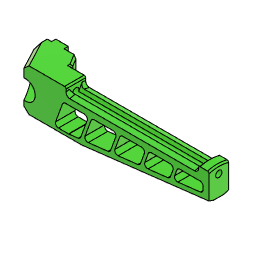
Single Piece Spool Holder v27 (Autodesk Fusion 360 design; units mm, degrees)
Autodesk Fusion 360 part; units mm, degrees
sketch "Sketch1" plane through (0, 0, 0) normal (0, 1, 0) x (1, 0, 0)
  line L0 (0, 0) -> (132, 0)
  line L1 (132, 0) -> (132, -30)
  line L2 (132, -30) -> (0, -30)
  line L3 (0, -30) -> (0, 0)
  line L4 (10, -30) -> (10, 0) construction
  line L5 (25, -30) -> (25, 0) construction
  dimension "d2" = 30
  dimension "d39" = 10
  dimension "d40" = 15
  dimension "d109" = 107
  constraint horizontal L0
  constraint vertical L1
  constraint horizontal L2
  constraint vertical L3
  constraint coincident L0.start L3.end
  constraint coincident L2 L4.start
  constraint coincident L0 L4.end
  constraint perpendicular L0 L4
  constraint coincident L2 L5.start
  constraint coincident L0 L5.end
  constraint perpendicular L0 L5
  measures "d2" distance of L0.start L2.end
  measures "d39" distance of L3 L4
  measures "d40" distance of L4 L5
  measures "d109" distance of L1 L5
extrude "Extrude1" add sketch "Sketch1" along normal mid plane 13 makes body 1
sketch "Sketch7" plane through (0, 6.5, 0) normal (0, 1, 0) x (-1, 0, 0)
  line L0 (0, 30) -> (-132, 30)
  line L1 (-132, 30) -> (-132, 0)
  line L2 (-132, 0) -> (0, 0)
  line L3 (0, 0) -> (0, 30)
  line L4 (0, 30) -> (-25, 30)
  line L5 (-25, 30) -> (-25, 0)
  line L6 (-25, 0) -> (0, 0)
  line L7 (0, 0) -> (0, 30)
  dimension "d75" = 25
  constraint horizontal L4
  constraint vertical L5
  constraint horizontal L6
  constraint vertical L7
  constraint coincident L2 L5.end
  constraint coincident L0.start L3.end
  measures "d75" distance of L0.start L4.end
extrude "Extrude9" add sketch "Sketch7" along normal blind 8.5 contours L0 L2 L3 L4 L5 L6 L7 bodies 1
sketch "Sketch2" plane through (0, 0, 0) normal (0, 0, 1) x (1, 0, 0)
  line L0 (0, -6.5) -> (0, 15)
  line L1 (25, 6.5) -> (132, 6.5)
  line L2 (132, 6.5) -> (132, -6.5)
  line L3 (132, -6.5) -> (0, -6.5)
  line L4 (5.825, 15) -> (14.175, 15)
  line L5 (14.175, 15) -> (14.175, 17.8)
  line L6 (14.175, 17.8) -> (5.825, 17.8)
  line L7 (5.825, 17.8) -> (5.825, 15)
  line L8 (10, 17.8) -> (10, 15) construction
  line L9 (0, 15) -> (25, 15)
  line L10 (25, 15) -> (25, 6.5)
  dimension "d20" = 10
  dimension "d21" = 2.8
  dimension "d22" = 8.35
  constraint horizontal L4
  constraint vertical L5
  constraint horizontal L6
  constraint vertical L7
  constraint midpoint L6 L8.start
  constraint midpoint L4 L8.end
  constraint coincident L9 L4.start
  constraint coincident L4.start L7.end
  measures "d20" distance of L0.end L8
  measures "d21" distance of L4.end L5.end
  measures "d22" distance of L5.end L6.end
extrude "Extrude2" add sketch "Sketch2" along normal blind 30 contours L4 L5 L6 L7 L9 bodies 1
sketch "Sketch3" plane through (0, -6.5, 0) normal (0, -1, 0) x (-1, 0, 0)
  line L0 (-10, -30) -> (-10, 0) construction
  circle A0 centre (-10, -15) radius 3.25
  line L1 (-132, -30) -> (0, -30)
  line L2 (0, -30) -> (0, 0)
  line L3 (0, 0) -> (-132, 0)
  line L4 (-132, 0) -> (-132, -30)
  line L5 (-14.175, 0) -> (-5.825, 0)
  line L6 (-5.825, 0) -> (-5.825, -30)
  line L7 (-5.825, -30) -> (-14.175, -30)
  line L8 (-14.175, -30) -> (-14.175, 0)
  dimension "d14" = 6.5
  constraint midpoint L0 A0.centre
  constraint midpoint L0.start L7
  constraint midpoint L0.end L5
  measures "d14" diameter of A0
extrude "Extrude3" cut sketch "Sketch3" against normal through all contours A0 bodies 1
sketch "Sketch4" plane through (0, -6.5, 0) normal (0, -1, 0) x (-1, 0, 0)
  circle A0 centre (-10, -15) radius 6.5
  circle A1 centre (-10, -15) radius 3.25
  line L0 (-132, -30) -> (0, -30)
  line L1 (0, -30) -> (0, 0)
  line L2 (0, 0) -> (-132, 0)
  line L3 (-132, 0) -> (-132, -30)
  dimension "d16" = 13
  constraint coincident A0.centre A1.centre
  measures "d16" diameter of A0
extrude "Extrude4" cut sketch "Sketch4" against normal up to surface (16 mm away) contours A0 | A1 bodies 1
chamfer "Chamfer1" distance 3.25 angle 45 1 edges at (13.0301, 9.5, 16.1753) on bodies 1
ref_plane "WorkPlane1" through (66, 5.65, 15) normal (0, 0, 1) x (1, 0, 0)
sketch "Sketch5" plane through (132, 0, 0) normal (1, 0, 0) x (0, 1, 0)
  line L0 (-6.5, 0) -> (6.5, 0)
  line L1 (6.5, 0) -> (6.5, 30)
  line L2 (6.5, 30) -> (-6.5, 30)
  line L3 (-6.5, 30) -> (-6.5, 0)
  circle A0 centre (0, 5.7) radius 20
  circle A1 centre (0, 5.7) radius 24
  line L4 (0, 0) -> (0, 30) construction
  circle A2 centre (0, 24.4) radius 2.1
  line L5 (-6.5, 0) -> (6.5, 0)
  line L6 (6.5, 0) -> (6.5, 30)
  line L7 (6.5, 30) -> (-6.5, 30)
  line L8 (-6.5, 30) -> (-6.5, 0)
  point P0 (27.1204, 5.059)
  point P1 (24.0412, 4.3321)
  point P2 (14.8796, 5.059)
  point P3 (17.9588, 4.3321)
  dimension "d86" = 40
  dimension "d87" = 48
  dimension "d88" = 5.7
  dimension "d89" = 24.4
  dimension "d90" = 4.2
  constraint coincident L4.start origin
  constraint midpoint L2 L4.end
  constraint coincident A0.centre A1.centre
  constraint coincident A0.centre L4
  constraint coincident L4 A2.centre
  measures "d86" diameter of A0
  measures "d87" diameter of A1
  measures "d88" distance of L0 A0.centre
  measures "d89" distance of L4.start A2.centre
  measures "d90" diameter of A2
extrude "Extrude5" cut sketch "Sketch5" against normal up to surface (88 mm away) from surface at -7 contours L1 L3 A0 A1 A2 L6 L8 | L1 L2 L3 A1 L6 L7 L8 | A0 A2 picked at (-0.0509, 25.9594) bodies 1
extrude "Extrude6" cut sketch "Sketch5" against normal blind 7 contours L1 L2 L3 A1 L6 L7 L8 bodies 1
extrude "Extrude7" cut sketch "Sketch5" against normal up to surface (102 mm away) contours A0 A2 | A0 A2 bodies 1
chamfer "Chamfer2" distance 1.3 distance2 2.2 2 edges at (81, -1.7041, 25.6273) (81, 1.7041, 25.6273) measured on face at (66.3333, -5.4581, 24.9408) measured on face at (66.3333, 2.2474, 25.5733) on bodies 1
fillet "Fillet1" radius 1 3 edges at (132, 0, 29.7) (125, 0, 29.7) (37, 0, 30) on bodies 1
chamfer "Chamfer3" distance 3 distance2 6 2 edges at (0, 4.25, 30) (0, 4.25, 0) measured on face at (20.3333, -2.1667, 30) measured on face at (52.3333, -2.1667, 0) on bodies 1
chamfer "Chamfer4" distance 11 distance2 93 1 edges at (132, 0, 0) measured on face at (132, 0.0523, 7.4353) on bodies 1
sketch "Sketch6" plane through (0, -6.5, 0) normal (0, -1, 0) x (1, 0, 0)
  line L0 (37, 24.6143) -> (37, 29)
  line L1 (36, 30) -> (3, 30)
  line L2 (3, 30) -> (0, 24)
  line L3 (0, 24) -> (0, 6)
  line L4 (0, 6) -> (3, 0)
  line L5 (3, 0) -> (39, 0)
  circle A0 centre (10, 15) radius 6.5
  line L6 (38.5445, 30) -> (27.6254, 0)
  line L7 (36.4161, 30) -> (25.497, 0)
  line L8 (0, 0) -> (128.5239, 0)
  line L9 (128.5239, 0) -> (128.5239, 30)
  line L10 (128.5239, 30) -> (0, 30)
  line L11 (0, 30) -> (0, 0)
  line L12 (55.4161, 30) -> (44.497, 0)
  line L13 (57.5445, 30) -> (46.6254, 0)
  line L14 (74.4161, 30) -> (63.497, 0)
  line L15 (76.5445, 30) -> (65.6254, 0)
  line L16 (93.4161, 30) -> (82.497, 0)
  line L17 (95.5445, 30) -> (84.6254, 0)
  line L18 (112.4161, 30) -> (101.497, 0)
  line L19 (114.5445, 30) -> (103.6254, 0)
  arc A1 (37, 29) -> (36, 30) centre (36, 29) ccw
  line L20 (39, 0) -> (132, 11)
  line L21 (132, 11) -> (132, 27.7624)
  spline S0 degree 3 poles (131, 28.803) (131.1219, 28.803) (131.2652, 28.7737) (131.4918, 28.6777) (131.6147, 28.5932) (131.7906, 28.4132) (131.8738, 28.285) (131.9704, 28.0461) (132, 27.8927) (132, 27.7624) knots 0.605058 0.605058 0.605058 0.605058 0.64162 0.64162 0.678904 0.678904 0.71712 0.71712 0.756197 0.756197 0.756197 0.756197
  line L22 (131, 28.803) -> (126, 28.803)
  spline S1 degree 3 poles (125, 27.7624) (125, 27.8927) (125.0296, 28.0461) (125.1262, 28.285) (125.2094, 28.4132) (125.3853, 28.5932) (125.5082, 28.6777) (125.7348, 28.7737) (125.8781, 28.803) (126, 28.803) knots 0.453919 0.453919 0.453919 0.453919 0.492996 0.492996 0.531212 0.531212 0.568496 0.568496 0.605058 0.605058 0.605058 0.605058
  line L23 (125, 27.7624) -> (125, 24.6143)
  line L24 (125, 24.6143) -> (37, 24.6143)
  line L25 (128, 14.5548) -> (128, 20.6143)
  line L26 (128, 20.6143) -> (33, 20.6143)
  line L27 (33, 20.6143) -> (33, 26)
  line L28 (33, 26) -> (5.4721, 26)
  line L29 (5.4721, 26) -> (4, 23.0557)
  line L30 (4, 23.0557) -> (4, 6.9443)
  line L31 (4, 6.9443) -> (5.4721, 4)
  line L32 (5.4721, 4) -> (38.7643, 4)
  line L33 (38.7643, 4) -> (128, 14.5548)
  line L34 (25, 30) -> (25, 0)
  line L35 (125, 22.6143) -> (35, 22.6143)
  line L36 (35, 22.6143) -> (35, 29)
  dimension "d51" = 2
  dimension "d55" = 76
  dimension "d56" = 0
  dimension "d59" = 30
  dimension "d61" = 70
  dimension "d101" = -4
  dimension "d108" = -2
  constraint parallel L6 L7
  constraint horizontal L8
  constraint vertical L9
  constraint horizontal L10
  constraint vertical L11
  constraint coincident L8.start L11.end
  constraint coincident L7.start L10
  constraint coincident L6.start L10
  constraint coincident L7.end L8
  constraint coincident L6.end L8
  constraint coincident L7 L26.end
  measures "d51" distance of L6 L7
  measures "d59" distance of L8 L10
  measures "d61" angle of L7 L10
extrude "Extrude8" cut sketch "Sketch6" against normal blind 47 contours L6 L12 L26 L32 L33 | L13 L14 L26 L33 | L15 L16 L26 L33 | L17 L18 L26 L33 | L19 L25 L26 L33 bodies 1
fillet "Fillet2" radius 2 21 edges at (35.1284, 0, 20.6143) (46.2763, 0, 4.8885) (68.3551, 0, 7.5) (85.9858, 0, 9.5853) (108.0647, 0, 12.1968) (128, 0, 14.5548) (128, 0, 20.6143) (111.1284, 0, 20.6143) (109, 0, 20.6143) (92.1284, 0, 20.6143) (90, 0, 20.6143) (73.1284, 0, 20.6143) (71, 0, 20.6143) (54.1284, 0, 20.6143) (52, 0, 20.6143) (38.7643, 0, 4) (48.5004, 0, 5.1516) (88.2099, 0, 9.8484) (105.8405, 0, 11.9338) (66.131, 0, 7.2369) (29.0813, 0, 4) on bodies 1
chamfer "Chamfer5" distance 3 distance2 1 2 edges at (85.5, -6.5, 5.5) (85.5, 6.5, 5.5) measured on face at (70, 2.1667, 3.6667) measured on face at (70, 2.1667, 3.6667) on bodies 1
chamfer "Chamfer6" distance 2 distance2 5 1 edges at (16.7433, -6.5, 0) measured on face at (27.0692, -6.5, 13.6608) on bodies 1
chamfer "Chamfer7" distance 9 distance2 17 1 edges at (0, -6.5, 15) measured on face at (27.0692, -6.5, 13.6608) on bodies 1
fillet "Fillet3" radius 2.5 4 edges at (37, -4.767, 25.1236) (37, 4.767, 25.1236) (125, -4.767, 25.1236) (125, 4.767, 25.1236) on bodies 1
chamfer "Chamfer12" distance 3 distance2 3 2 edges at (6, -0.8333, 30) (7.6765, -4, 1) measured on face at (6.2596, -1.3237, 26.8819) measured on face at (6.2596, -1.3237, 26.8819) on bodies 1
sketch "Sketch8" plane through (0, 17.8, 0) normal (0, 1, 0) x (-1, 0, 0)
  circle A0 centre (-10, 15) radius 3.25
  line L0 (-14.175, 0) -> (-5.825, 0)
  line L1 (-5.825, 0) -> (-5.825, 30)
  line L2 (-5.825, 30) -> (-14.175, 30)
  line L3 (-14.175, 30) -> (-14.175, 0)
  line L4 (-5.825, 22.5) -> (-14.175, 22.5)
  line L5 (-14.175, 22.5) -> (-14.175, 7.5)
  line L6 (-14.175, 7.5) -> (-5.825, 7.5)
  line L7 (-5.825, 7.5) -> (-5.825, 22.5)
  line L8 (-5.825, 22.5) -> (-14.175, 7.5) construction
  line L9 (-14.175, 22.5) -> (-5.825, 7.5) construction
  point P0 (-10, 15)
  dimension "d93" = 15
  constraint horizontal L4
  constraint perpendicular L4 L5
  constraint parallel L4 L6
  constraint parallel L5 L7
  constraint coincident L1 L4.start
  constraint coincident L8 P0
  constraint coincident L9 P0
  constraint coincident P0 A0.centre
  measures "d93" distance of L4.start L6.end
extrude "Extrude10" cut sketch "Sketch8" against normal up to surface (2.8 mm away) contours L1 L3 L4 L5 L6 L7 bodies 1
sketch "Sketch9" plane through (132, 0, 0) normal (1, 0, 0) x (0, 1, 0)
  arc A0 (6.5, 27.7624) -> (-6.5, 27.7624) centre (0, 5.7) ccw
  circle A1 centre (0, 24.4) radius 2
  circle A2 centre (0, 24.4) radius 1
  line L0 (3.5, 11) -> (6.5, 12.007)
  line L1 (6.5, 12.007) -> (6.5, 27.7624)
  line L2 (-6.5, 27.7624) -> (-6.5, 12.007)
  line L3 (-6.5, 12.007) -> (-3.5, 11)
  line L4 (-3.5, 11) -> (3.5, 11)
  circle A3 centre (0, 24.4) radius 2.1
  dimension "d96" = 4
  dimension "d97" = 2
  measures "d96" diameter of A1
  measures "d97" diameter of A2
extrude "Extrude11" add sketch "Sketch9" against normal blind 100.25 separate body contours A1 makes body 2
chamfer "Chamfer13" distance 3 distance2 5 1 edges at (25, 15, 15) measured on face at (21.0833, 15, 15) on bodies 1
chamfer "Chamfer14" distance 2 distance2 1 2 edges at (23.5, 12.5, 30) (23.5, 12.5, 0) measured on face at (24, 11.6667, 20) measured on face at (24, 11.6667, 20) on bodies 1
move_body "Move1" [suppressed]
hidden bodies 2
named bodies: "Single Piece Spool Holder"
